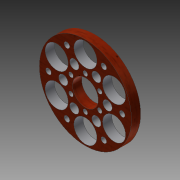
# Autodesk Inventor part: Статор цевков
Saved by Autodesk Inventor 2013 (Build 170138000, 138)
## iProperties
Created: 2014-04-30
Part Number: Статор цевков
Material: Типовые
Document SubType Name: Modeling
Designer: HP1
Density: 1 g/cm^3
Author: HP1
Autodesk Inventor part; units mm, degrees
ref_plane "YZ Plane" through (0, 0, 0) normal (1, 0, 0) x (0, 1, 0)
ref_plane "XZ Plane" through (0, 0, 0) normal (0, 1, 0) x (-1, 0, 0)
ref_plane "XY Plane" through (0, 0, 0) normal (0, 0, 1) x (1, 0, 0)
sketch "Эскиз1" plane through (0, 0, 0) normal (0, 1, 0) x (-1, 0, 0)
  circle A0 centre (0, 0) radius 14
  circle A1 centre (0, 0) radius 24 construction
  circle A2 centre (0, 0) radius 50
  circle A3 centre (23.9999, 0) radius 5
  circle A4 centre (12, 20.7845) radius 5
  circle A5 centre (-12, 20.7845) radius 5
  circle A6 centre (-23.9999, 0) radius 5
  circle A7 centre (-12, -20.7845) radius 5
  circle A8 centre (12, -20.7845) radius 5
  dimension "d0" = 28
  dimension "d1" = 48
  dimension "d2" = 100
  dimension "d3" = 10
  dimension "d6" = 360
  constraints: 9 centre point, 13 other
  measures "d0" diameter of A0
  measures "d1" diameter of A1
  measures "d2" diameter of A2
  measures "d3" diameter of A3
extrude "Выдавливание1" add sketch "Эскиз1" along normal blind 10
sketch "Эскиз2" plane through (0, 10, 0) normal (0, 1, 0) x (1, 0, 0)
  circle A0 centre (0, 0) radius 14 projected
  circle A1 centre (0, 36) radius 12.5
  circle A2 centre (-31.1769, 18) radius 12.5
  circle A3 centre (-31.1769, -18) radius 12.5
  circle A4 centre (0, -36) radius 12.5
  circle A5 centre (31.1769, -18) radius 12.5
  circle A6 centre (31.1769, 18) radius 12.5
  dimension "d10" = 25
  dimension "d13" = 360
  dimension "d19" = 36
  constraints: 6 centre point, 13 other
  measures "d10" diameter of A1
  measures "d19" distance of A0.centre A1.centre
extrude "Выдавливание2" cut sketch "Эскиз2" against normal blind 10 contours A1 | A2 | A3 | A4 | A5 | A6
sketch "Эскиз3" plane through (0, 10, 0) normal (0, 1, 0) x (1, 0, 0)
  circle A0 centre (0, 0) radius 50 projected
  circle A1 centre (0, 0) radius 14 projected
  circle A2 centre (0, 18) radius 2.5
  circle A3 centre (-15.5885, 9) radius 2.5
  circle A4 centre (-15.5885, -9) radius 2.5
  circle A5 centre (0, -18) radius 2.5
  circle A6 centre (15.5885, -9) radius 2.5
  circle A7 centre (15.5885, 9) radius 2.5
  point P0 (22.396, 26.8964)
  point P1 (12.095, 32.8438)
  dimension "d20" = 5
  dimension "d22" = 18
  dimension "d25" = 360
  constraints: 6 centre point, 14 other
  measures "d20" diameter of A2
  measures "d22" distance of point (0, 0) A2.centre
extrude "Выдавливание3" cut sketch "Эскиз3" against normal blind 10 contours A2 | A3 | A4 | A5 | A6 | A7
sketch "Эскиз4" plane through (0, 10, 0) normal (0, 1, 0) x (1, 0, 0)
  circle A0 centre (0, 0) radius 14 projected
  circle A1 centre (40, 0) radius 3
  circle A2 centre (20, 34.641) radius 3
  circle A3 centre (-20, 34.641) radius 3
  circle A4 centre (-40, 0) radius 3
  circle A5 centre (-20, -34.641) radius 3
  circle A6 centre (20, -34.641) radius 3
  dimension "d29" = 6
  dimension "d30" = 40
  dimension "d33" = 360
  constraints: 6 centre point, 13 other
  measures "d29" diameter of A1
  measures "d30" distance of A0.centre A1.centre
extrude "Выдавливание4" cut sketch "Эскиз4" against normal blind 10 contours A1 | A2 | A3 | A4 | A5 | A6
